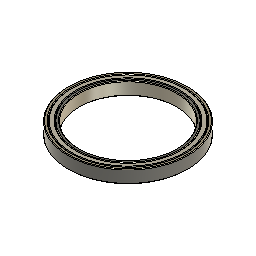
Epaule (Autodesk Fusion 360 archive; units mm, degrees)
design "Roullement 30x37x4"
Autodesk Fusion 360 part; units mm, degrees
sketch "Sketch1" plane through (0, 0, 0) normal (0, 0, 1) x (1, 0, 0)
  circle A0 centre (0, 0) radius 18.5
  circle A1 centre (0, 0) radius 15
  circle A2 centre (0, 0) radius 17.5
  circle A3 centre (0, 0) radius 16
  dimension "d1" = 37
  dimension "d2" = 30
  dimension "d5" = -1
  dimension "d6" = 1
  constraint coincident A0.centre A1.centre
  measures "d1" diameter of A0
  measures "d2" diameter of A1
extrude "Extrude2" add sketch "Sketch1" along normal blind 4 contours A0 makes body 1
fillet "Fillet1" radius 0.2 2 edges at (-17.2481, -6.6899, 4) (-16.3157, 6.3283, 4) on bodies 1
fillet "Fillet1" radius 0.2 2 edges at (-17.2481, -6.6899, 0) (-16.3157, 6.3283, 0) on bodies 1
extrude "Extrude3" add sketch "Sketch1" along normal blind 4 separate body contours A3 makes body 2
fillet "Fillet2" radius 0.2 2 edges at (-14.9172, -5.7858, 4) (-13.9849, 5.4242, 4) on bodies 2
fillet "Fillet2" radius 0.2 2 edges at (-14.9172, -5.7858, 0) (-13.9849, 5.4242, 0) on bodies 2
extrude "Extrude4" add sketch "Sketch1" along normal blind 4 separate body contours A2 makes body 3
fillet "Fillet3" radius 0.2 2 edges at (-16.3157, -6.3283, 4) (-14.9172, 5.7858, 4) on bodies 3
fillet "Fillet3" radius 0.2 2 edges at (-16.3157, -6.3283, 0) (-14.9172, 5.7858, 0) on bodies 3
combine "Combine1" operation add target body 1 tool bodies 2 3

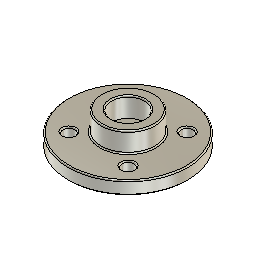
design "Servo ARM"
Autodesk Fusion 360 part; units mm, degrees
sketch "Sketch1" plane through (0, 0, 0) normal (0, 0, 1) x (-1, 0, 0) in component "Servo ARM"
  circle A0 centre (0, 0) radius 2.75
  circle A1 centre (0, 0) radius 4.5
  circle A2 centre (0, 0) radius 1.5
  circle A3 centre (0, 0) radius 2.1
  circle A4 centre (0, 0) radius 10
  line L0 (-4.9497, 4.9497) -> (4.9497, 4.9497) construction
  line L1 (4.9497, 4.9497) -> (4.9497, -4.9497) construction
  line L2 (4.9497, -4.9497) -> (-4.9497, -4.9497) construction
  line L3 (-4.9497, -4.9497) -> (-4.9497, 4.9497) construction
  line L4 (-4.9497, 4.9497) -> (4.9497, -4.9497) construction
  line L5 (4.9497, 4.9497) -> (-4.9497, -4.9497) construction
  circle A5 centre (4.9497, -4.9497) radius 1
  circle A6 centre (-4.9497, -4.9497) radius 1
  circle A7 centre (4.9497, 4.9497) radius 1
  circle A8 centre (-4.9497, 4.9497) radius 1
  circle A9 centre (0, 0) radius 7
  dimension "d18_1" = 5.5
  dimension "d19_1" = 9
  dimension "d20_1" = 3
  dimension "d1" = 20
  dimension "d2" = 2
  dimension "d3" = 2
  dimension "d4" = 2
  dimension "d5" = 2
  dimension "d7" = 14
  constraint concentric A0 A1
  constraint coincident A0.centre A1.centre
  constraint concentric A1 A4
  constraint horizontal L0
  constraint perpendicular L0 L1
  constraint parallel L0 L2
  constraint parallel L1 L3
  constraint coincident L4 A0.centre
  constraint coincident L5 A0.centre
  constraint coincident L1.end L2.start
  constraint coincident L2.end L3.start
  constraint coincident L0.end L1.start
  constraint coincident L0.start L3.end
  constraint concentric A4 A9
  constraint coincident L2.end A9
  constraint equal L0 L1
  measures "d18_1" diameter of A0
  measures "d19_1" diameter of A1
  measures "d20_1" diameter of A2
  measures "d1" diameter of A4
  measures "d2" diameter of A5
  measures "d3" diameter of A6
  measures "d4" diameter of A7
  measures "d5" diameter of A8
  measures "d7" diameter of A9
extrude "Extrude1" add sketch "Sketch1" along normal blind 2.2 contours A0 | A3 | A4 | A5 A6 A7 A8 A9 makes body 1 at (2.45, 6.5498, 0) makes body 2 at (-2.7363, 0.2738, 1.4667) in component "Servo ARM"
extrude "Extrude2" add sketch "Sketch1" along normal blind 5.5 contours A1 bodies 1 2 in component "Servo ARM"
fillet "Fillet1" radius 0.2 1 faces at (2.45, 6.5498, 2.2) on bodies 1 in component "Servo ARM"
fillet "Fillet2" radius 0.2 1 faces at (0.2491, 6.7232, 0) on bodies 1 in component "Servo ARM"
fillet "Fillet3" radius 0.2 1 faces at (-3.8897, 0.3602, 5.5) on bodies 1 in component "Servo ARM"
component "Servo ARM" placed x (1, 0, 0) y (0, 1, 0) z (0, 0, 1) at (0, 0, 0)
